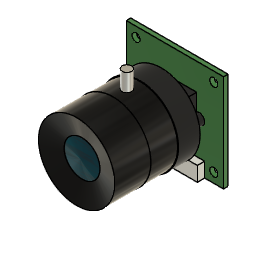
Arducam OV5647 v1 (Autodesk Fusion 360 design; units mm, degrees)
Autodesk Fusion 360 part; units mm, degrees
sketch "Body" plane through (0, 0, 0) normal (0, 1, 0) x (1, 0, 0)
  line L0 (18, 18) -> (-18, 18)
  line L1 (-18, 18) -> (-18, -18)
  line L2 (-18, -18) -> (18, -18)
  line L3 (18, -18) -> (18, 18)
  line L4 (18, 18) -> (-18, -18) construction
  line L5 (-18, 18) -> (18, -18) construction
  dimension "d1" = 36
  dimension "d2" = 36
  constraint horizontal L0
  constraint perpendicular L0 L1
  constraint parallel L0 L2
  constraint parallel L1 L3
  constraint coincident L4 origin
  constraint coincident L5 origin
  measures "d1" distance of L1.end L2.end
  measures "d2" distance of L0.end L1.end
extrude "Extrude1" add sketch "Body" along normal blind 1.65 makes body 1
sketch "Mounting Holes" plane through (0, 0, 0) normal (0, -1, 0) x (1, 0, 0)
  line L0 (18, -18) -> (18, 18)
  line L1 (18, 18) -> (-18, 18)
  line L2 (-18, 18) -> (-18, -18)
  line L3 (-18, -18) -> (18, -18)
  point P0 (-14.4, 14.4)
  point P1 (14.4, 14.4)
  point P2 (-14.4, -14.4)
  point P3 (14.4, -14.4)
  dimension "d7" = 28.8
  dimension "d8" = -28.8
  dimension "d9" = 3.6
  dimension "d10" = 3.6
  measures "d9" distance of L1 P0
  measures "d10" distance of L2 P0
hole "Hole1" at (-14.4, 0, 14.4) at (14.4, 0, 14.4) at (14.4, 0, -14.4) at (-14.4, 0, -14.4) direction (0, 1, 0) diameter 3 end through all bodies 1
sketch "Sensor" plane through (0, 0, 0) normal (0, -1, 0) x (1, 0, 0)
  circle A0 centre (14.4, -14.4) radius 1.5
  circle A1 centre (-14.4, 14.4) radius 1.5
  circle A2 centre (14.4, 14.4) radius 1.5
  circle A3 centre (-14.4, -14.4) radius 1.5
  line L0 (18, -18) -> (18, 18)
  line L1 (18, 18) -> (-18, 18)
  line L2 (-18, 18) -> (-18, -18)
  line L3 (-18, -18) -> (18, -18)
  line L4 (8.05, -8.05) -> (-8.05, -8.05)
  line L5 (-8.05, 8.05) -> (8.05, 8.05)
  line L6 (8.05, -8.05) -> (-8.05, 8.05) construction
  line L7 (-8.05, -8.05) -> (8.05, 8.05) construction
  line L8 (-15, 0) -> (15, 0) construction
  arc A4 (-8.05, 1.76) -> (-8.05, -1.76) centre (-9, 0) ccw
  line L9 (-8.05, -8.05) -> (-8.05, -1.76)
  line L10 (-8.05, 1.76) -> (-8.05, 8.05)
  line L11 (8.05, 8.05) -> (8.05, 1.76)
  line L12 (8.05, -1.76) -> (8.05, -8.05)
  arc A5 (8.05, -1.76) -> (8.05, 1.76) centre (9, 0) ccw
  dimension "d14" = 16.1
  dimension "d15" = 16.1
  dimension "d17" = 4
  dimension "d18" = 4
  dimension "d19" = 9
  dimension "d20" = 9
  constraint horizontal L4
  constraint perpendicular L4 L9
  constraint parallel L4 L5
  constraint parallel L9 L11
  constraint coincident L6 origin
  constraint coincident L7 origin
  constraint perpendicular L8 L11
  constraint coincident origin L8
  constraint coincident A4.centre L8
  constraint coincident A5.centre L8
  constraint coincident A4.start L9
  constraint collinear L9 L10
  constraint collinear L11 L12
  measures "d14" distance of L5.start L5.end
  measures "d15" distance of L4.end L5.start
  measures "d17" diameter of A4
  measures "d18" diameter of A5
  measures "d19" distance of origin A4.centre
  measures "d20" distance of origin A5.centre
extrude "Extrude2" add sketch "Sensor" along normal blind 5 separate body contours L4 L5 A4 L9 L10 L11 L12 A5 makes body 2
sketch "Lens1" plane through (0, -5, 0) normal (0, -1, 0) x (1, 0, 0)
  line L0 (8.05, -8.05) -> (8.05, -1.76)
  arc A0 (8.05, -1.76) -> (8.05, 1.76) centre (9, 0) ccw
  line L1 (8.05, 1.76) -> (8.05, 8.05)
  line L2 (8.05, 8.05) -> (-8.05, 8.05)
  line L3 (-8.05, 8.05) -> (-8.05, 1.76)
  arc A1 (-8.05, 1.76) -> (-8.05, -1.76) centre (-9, 0) ccw
  line L4 (-8.05, -1.76) -> (-8.05, -8.05)
  line L5 (-8.05, -8.05) -> (8.05, -8.05)
  circle A2 centre (0, 0) radius 14.3
  dimension "d24" = 28.6
  constraint coincident A2.centre origin
  measures "d24" diameter of A2
extrude "Extrude3" add sketch "Lens1" along normal blind 8 separate body contours L0 A0 L1 L2 L3 A1 L4 L5 | A2 makes body 3
sketch "Lens2" plane through (0, -13, 0) normal (0, -1, 0) x (1, 0, 0)
  circle A0 centre (0, 0) radius 14
  circle A1 centre (0, 0) radius 14.3
  dimension "d28" = 28
  constraint coincident A0.centre A1.centre
  measures "d28" diameter of A0
extrude "Extrude5" add sketch "Lens2" along normal blind 10 separate body contours A0 makes body 4
sketch "Lens3" plane through (0, -23, 0) normal (0, -1, 0) x (1, 0, 0)
  circle A0 centre (0, 0) radius 14.1
  circle A1 centre (0, 0) radius 14
  dimension "d34" = 28.2
  constraint coincident A0.centre A1.centre
  measures "d34" diameter of A0
extrude "Extrude6" add sketch "Lens3" along normal blind 13.4 separate body contours A0 | A1 makes body 5
ref_plane "WorkPlane3" through (0, -19.1055, 14) normal (0, 0, 1) x (1, 0, 0)
sketch "Focus Lock" plane through (0, -19.3055, 14) normal (0, 0, 1) x (1, 0, 0)
  circle A0 centre (0, 1.5) radius 1.75
  dimension "d41" = 3.5
  dimension "d42" = 1.5
  measures "d41" diameter of A0
  measures "d42" distance of origin A0.centre
extrude "Extrude7" add sketch "Focus Lock" along normal blind 6.5 separate body makes body 6
sketch "Connector" plane through (0, 0, 0) normal (0, -1, 0) x (1, 0, 0)
  circle A0 centre (14.4, -14.4) radius 1.5
  circle A1 centre (-14.4, 14.4) radius 1.5
  circle A2 centre (14.4, 14.4) radius 1.5
  circle A3 centre (-14.4, -14.4) radius 1.5
  line L0 (18, -18) -> (18, 18)
  line L1 (18, 18) -> (-18, 18)
  line L2 (-18, 18) -> (-18, -18)
  line L3 (-18, -18) -> (18, -18)
  line L4 (-11, -18) -> (11, -18)
  line L5 (11, -18) -> (11, -12.6)
  line L6 (11, -12.6) -> (-11, -12.6)
  line L7 (-11, -12.6) -> (-11, -18)
  dimension "d43" = 22
  dimension "d44" = 5.4
  dimension "d45" = 7
  constraint horizontal L4
  constraint vertical L5
  constraint horizontal L6
  constraint vertical L7
  constraint coincident L3 L4.start
  measures "d43" distance of L4.start L4.end
  measures "d44" distance of L4.start L6.end
  measures "d45" distance of L0 L5
extrude "Extrude8" add sketch "Connector" along normal blind 2.7 separate body contours L3 L4 L5 L6 L7 makes body 7
extrude "Extrude9" cut 1 faces at (-0.3512, -36.4, 3.4538) along direction (0, 1, 0) blind 2 draft -75 on bodies 5 bodies 5
sketch "Front Lens" plane through (0, -34.4, 0) normal (0, -1, 0) x (1, 0, 0)
  circle A0 centre (0, 0) radius 6.6359
extrude "Extrude10" add sketch "Front Lens" along normal blind 0.6 draft -85 separate body makes body 8
equation "d18 = d17"
equation "d20 = d19"
named bodies: "Sensor", "Lens1", "Lens2", "Lens3", "Focus Lock", "Connector", "Front Lens"
